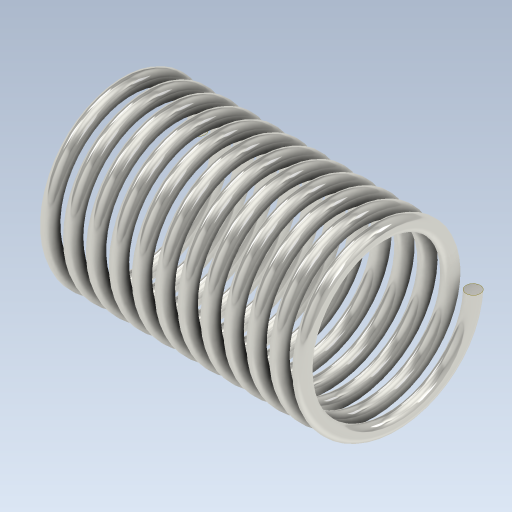
# Autodesk Inventor part: resorte
Saved by Autodesk Inventor 2023 (Build 270158000, 158)
## iProperties
Created: 2023-03-26
Part Number: resorte
Material: Silver
Document SubType Name: Modeling
Designer: santi
Density: 10.49 g/cm^3
Appearance: Silver
Author: santi
Autodesk Inventor part; units mm, degrees
ref_plane "YZ Plane" through (0, 0, 0) normal (1, 0, 0) x (0, 1, 0)
ref_plane "XZ Plane" through (0, 0, 0) normal (0, 1, 0) x (-1, 0, 0)
ref_plane "XY Plane" through (0, 0, 0) normal (0, 0, 1) x (1, 0, 0)
sketch "Sketch2" plane through (0, 0, 0) normal (0, 1, 0) x (-1, 0, 0)
  circle A0 centre (0, -5.5) radius 0.5
  point P0 (0, 0)
  dimension "d0" = 1
  dimension "d1" = 5.5
  constraints: 1 centre point, 1 vertical alignment
  measures "d0" diameter of A0
  measures "d1" distance of A0.centre point (0, 0)
coil "Coil1" sketch "Sketch2" operation add axis through (-10, 0, 0) along (1, 0, 0) pitch 1.5833 turns 12 hand right
body "Solid1"
